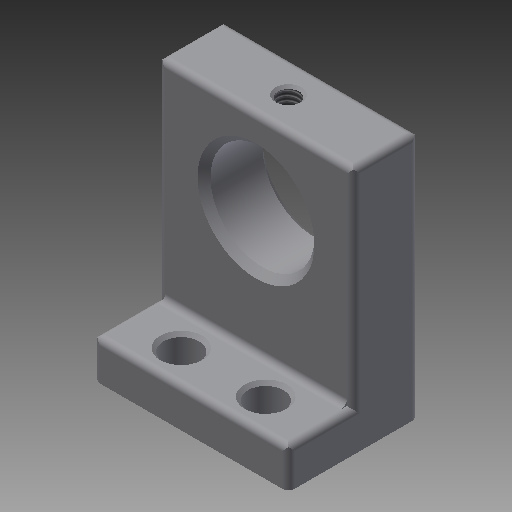
# Autodesk Inventor part: SHKLMT16b
Saved by Autodesk Inventor 2019 (Build 230136000, 136)
## iProperties
Category: PARTsolutions
Company: MISUMI
Created: 2019-04-24
Part Number: SHKLMT16b
Material: 일반
Catalog Web Link: www.cadenas.de
Description: SHKLBT, SHKLMT, SHKLST-b-Shaft Supports - Casting - L-Shaped - Standard
Vendor: MISUMI
Document SubType Name: Modeling
Designer: psadmin
Manufacturer: MISUMI
Mass: 10.6619 g
Surface Area: 44.4206 cm^2
Volume: 10.6619 cm^3
Density: 1 g/cm^3
Appearance: PSOLRGB-192-192-192
PSOL_IDENT_0: {$CADENAS_DATA\23d-libs\misumi\metric\02_shaft_supports\shklbt_b.prj},174 {VTYP=3D},{NB=SHKLMT16b},{
PSOL_IDENT_1: LINA=SHKLMT16b},{NN=SHKLBT, SHKLMT, SHKLST-b},{DATE=30.03.2018 01:12:39},{GEOMDATE=14.04.2006},{VERS
PSOL_IDENT_2: ION=},{LINEID=100},{WBVAR=MAT,ST},{WBNUMERIC=}  {NB=SHKLMT16b},{LINA=SHKLMT16b},{KT=DUMMY},{PN=SHKLM
PSOL_IDENT_3: T16},{TYPE=SHKLMT},{MAT=1045},{ST=Electroless Nickel Plating},{AC=Set Screw 1 Pc.},{D=16},{H=25},{L=
PSOL_IDENT_4: 30},{H1=38},{T=10},{S=6},{W=20},{W1=15},{A=12.5},{M=M4 },{L1=13},{DD=5.5},{ST0='Black Oxide','Black
PSOL_IDENT_5: Oxide','Electroless Nickel Plating','Electroless Nickel Plating'},{B1=14},{B2=8},{B3=2},{MASS=79},{T
PSOL_IDENT_6: HMD=4},{THDMIN=3.242},{LM=6},{MASSS=79},{MASSA=28}
NN: SHKLBT, SHKLMT, SHKLST-b
NT: Shaft Supports - Casting - L-Shaped - Standard
NB: SHKLMT16b
NBSYN: $PN.b
LINA: SHKLMT16b
PN: SHKLMT16
MAT: 1045 Steel
ST: Electroless Nickel Plating
AC: Set Screw 1 Pc.
D: 16
H: 25
L: 30
H1: 38
T: 10
S: 6
W: 20
W1: 15
A: 12.5
M: M4
L1: 13
DD: 5.5
B1: 14
B2: 8
B3: 2
SUPPLIER: MISUMI
ARTICLENO: SHKLMT16b
BOMINFO: SHKLMT16b
CREATOR: CADENAS GmbH
Title: SHKLMT16b
Author: Cadenas PARTsolutions
Comments: Shaft Supports - Casting - L-Shaped - Standard
Autodesk Inventor part; units mm, degrees
sketch "Sketch_9" plane through (0, 0, 0) normal (0, 0, 1) x (1, 0, 0)
  line L0 (-15, 5) -> (-15, 0)
  line L1 (-15, 0) -> (15, 0)
  line L2 (15, 0) -> (15, 5)
  arc A0 (15, 5) -> (14, 6) centre (14, 5) ccw
  line L3 (14, 6) -> (-14, 6)
  arc A1 (-14, 6) -> (-15, 5) centre (-14, 5) ccw
  constraints: 8 end point, 4 point on circle, 2 centre point
sketch "Sketch_10" plane through (0, 0, 0) normal (0, 1, 0) x (-1, 0, 0)
  line L0 (15, 1) -> (15, 9)
  arc A0 (15, 9) -> (14, 10) centre (14, 9) ccw
  line L1 (14, 10) -> (-14, 10)
  arc A1 (-14, 10) -> (-15, 9) centre (-14, 9) ccw
  line L2 (-15, 9) -> (-15, 1)
  arc A2 (-15, 1) -> (-14, 0) centre (-14, 1) ccw
  line L3 (-14, 0) -> (14, 0)
  arc A3 (14, 0) -> (15, 1) centre (14, 1) ccw
  constraints: 8 end point, 8 point on circle, 4 centre point
extrude "Extrusion1" add sketch "Sketch_9" along normal blind 20
extrude "Extrusion2" add sketch "Sketch_10" along normal blind 38
sketch "Sketch_5" plane through (0, 0, 0) normal (0, 0, 1) x (1, 0, 0)
  arc A0 (-14, 38) -> (-15, 37) centre (-14, 37) ccw
  line L0 (-14, 38) -> (14, 38)
  arc A1 (15, 37) -> (14, 38) centre (14, 37) ccw
  line L1 (15, 37) -> (15, 76)
  line L2 (15, 76) -> (-15, 76)
  line L3 (-15, 76) -> (-15, 37)
  constraints: 8 end point, 4 point on circle, 2 centre point
extrude "Extrusion3" cut sketch "Sketch_5" along normal blind 10
sketch "Sketch_7" plane through (0, 0, 0) normal (1, 0, 0) x (0, 1, 0)
  line L0 (25, 0) -> (25, 10)
  line L1 (25, 10) -> (34, 10)
  line L2 (34, 10) -> (33, 9)
  line L3 (33, 9) -> (33, 1)
  line L4 (33, 1) -> (34, 0)
  line L5 (34, 0) -> (25, 0)
  line L6 (25, 0) -> (25, 10)
  constraints: 14 end point
revolve "Revolution1" cut sketch "Sketch_7" angle 360 about axis through (0, 25, 0) along (0, 0, -1)
sketch "Sketch_1" plane through (0, 0, 5) normal (0, 0, 1) x (1, 0, 0)
  line L0 (0, 25) -> (0, 38)
  line L1 (0, 38) -> (2, 38)
  line L2 (2, 38) -> (1.621, 37.621)
  line L3 (1.621, 37.621) -> (1.621, 33)
  line L4 (1.621, 33) -> (2, 32.621)
  line L5 (2, 32.621) -> (2, 25)
  line L6 (2, 25) -> (0, 25)
  line L7 (0, 25) -> (0, 38)
  constraints: 16 end point
revolve "Revolution2" cut sketch "Sketch_1" angle 360 about axis through (0, 25, 5) along (0, -1, 0)
thread "Thread1" size "M4x0.7" class "6H" standard "ISO Metric profile" full length
sketch "Sketch6" plane through (-14, 6, 20) normal (0, 1, 0) x (1, 0, 0)
  point P0 (7.5, 5)
hole "Hole1" at (-6.5, 6, 15) direction (0, -1, 0) diameter 5.5 depth 6 countersink diameter 6.5 countersink angle 90
sketch "Sketch7" plane through (-14, 6, 20) normal (0, 1, 0) x (1, 0, 0)
  point P0 (20.5, 5)
hole "Hole2" at (6.5, 6, 15) direction (0, -1, 0) diameter 5.5 depth 6 countersink diameter 6.5 countersink angle 90
sketch "Sketch_4" plane through (0, 0, 0) normal (0, 1, 0) x (-1, 0, 0)
  line L0 (30, -10) -> (30, 30)
  line L1 (30, 30) -> (-30, 30)
  line L2 (-30, 30) -> (-30, -10)
  line L3 (-30, -10) -> (30, -10)
  line L4 (15, 1) -> (15, 19)
  arc A0 (15, 19) -> (14, 20) centre (14, 19) ccw
  line L5 (14, 20) -> (-14, 20)
  arc A1 (-14, 20) -> (-15, 19) centre (-14, 19) ccw
  line L6 (-15, 19) -> (-15, 1)
  arc A2 (-15, 1) -> (-14, 0) centre (-14, 1) ccw
  line L7 (-14, 0) -> (14, 0)
  arc A3 (14, 0) -> (15, 1) centre (14, 1) ccw
  constraints: 16 end point, 8 point on circle, 4 centre point
extrude "Extrusion4" cut sketch "Sketch_4" along normal blind 38
sketch "Sketch_8" plane through (0, 0, 0) normal (0, 0, 1) x (1, 0, 0)
  line L0 (-7, 10) -> (-7, 2)
  line L1 (-7, 2) -> (7, 2)
  line L2 (7, 2) -> (7, 10)
  line L3 (7, 10) -> (-7, 10)
  constraints: 8 end point
extrude "Extrusion5" cut sketch "Sketch_8" along normal blind 0.8
sketch "Sketch_6" plane through (0, 0, 0) normal (1, 0, 0) x (0, 1, 0)
  line L0 (57, 30) -> (-19, 30)
  line L1 (-19, 30) -> (-19, -10)
  line L2 (-19, -10) -> (57, -10)
  line L3 (57, -10) -> (57, 30)
  line L4 (5, 20) -> (0, 20)
  line L5 (0, 20) -> (0, 0)
  line L6 (0, 0) -> (37, 0)
  arc A0 (37, 0) -> (38, 1) centre (37, 1) ccw
  line L7 (38, 1) -> (38, 9)
  arc A1 (38, 9) -> (37, 10) centre (37, 9) ccw
  line L8 (37, 10) -> (6, 10)
  line L9 (6, 10) -> (6, 19)
  arc A2 (6, 19) -> (5, 20) centre (5, 19) ccw
  constraints: 20 end point, 6 point on circle, 3 centre point
extrude "Extrusion6" cut sketch "Sketch_6" along normal mid plane 30
sketch "Sketch_11" plane through (0, 0, 0) normal (1, 0, 0) x (0, 1, 0)
  line L0 (6, 11) -> (3, 11)
  line L1 (3, 11) -> (3, 5)
  line L2 (3, 5) -> (7, 5)
  line L3 (7, 5) -> (7, 10)
  arc A0 (6, 11) -> (7, 10) centre (7, 11) ccw
  constraints: 8 end point, 2 point on circle, 1 centre point
extrude "Extrusion7" add sketch "Sketch_11" along normal mid plane 28
ref_plane "b_s_XY" through (0, 38, 5) normal (0, 1, 0) x (1, 0, 0)
ref_plane "b_s_YZ" through (0, 38, 5) normal (1, 0, 0) x (0, 0, -1)
ref_plane "b_s_ZX" through (0, 38, 5) normal (0, 0, -1) x (0, 1, 0)
body "Solid1"
